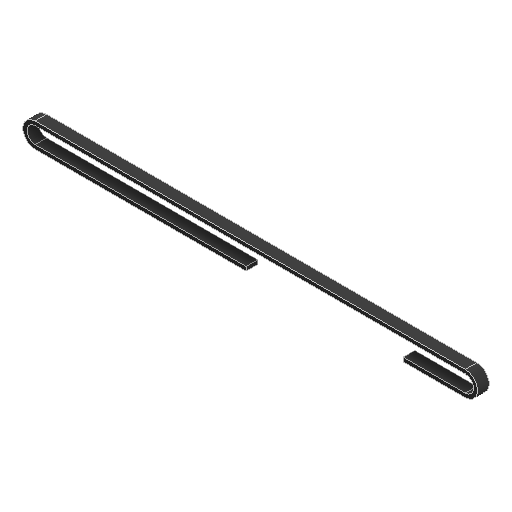
# Autodesk Inventor part: Riemen_T5
Saved by Autodesk Inventor 2022 (Build 260153000, 153)
## iProperties
Created: 2022-10-06
Part Number: Riemen_T5
Material: Gummi
Document SubType Name: Modeling
Designer: alexw
Mass: 23.1241 g
Surface Area: 192.513 cm^2
Volume: 24.8646 cm^3
Density: 0.93 g/cm^3
Appearance: Gummi - Schwarz
Author: alexw
Autodesk Inventor part; units mm, degrees
ref_plane "YZ Plane" through (0, 0, 0) normal (1, 0, 0) x (0, 1, 0)
ref_plane "XZ Plane" through (0, 0, 0) normal (0, 1, 0) x (-1, 0, 0)
ref_plane "XY Plane" through (0, 0, 0) normal (0, 0, 1) x (1, 0, 0)
sketch "Skizze1" plane through (0, 0, 0) normal (0, 0, 1) x (1, 0, 0)
  circle A0 centre (-380.4963, -115.5552) radius 3 construction
  circle A1 centre (-10.4963, -115.5552) radius 3.1 construction
  circle A2 centre (-380.4963, -115.5552) radius 10.57 construction
  circle A3 centre (-10.4963, -115.5552) radius 10.57 construction
  line L0 (-10.4963, -104.9852) -> (-380.4963, -104.9852)
  line L1 (-380.4963, -115.5552) -> (-380.4963, -104.9852) construction
  arc A4 (-380.4963, -104.9852) -> (-380.4963, -126.1252) centre (-380.4963, -115.5552) ccw
  line L2 (-380.4963, -126.1252) -> (-10.4963, -126.1252)
  arc A5 (-10.4963, -126.1252) -> (-10.4963, -104.9852) centre (-10.4963, -115.5552) ccw
  circle A6 centre (-380.4963, -115.5552) radius 7.07 construction
  circle A7 centre (-10.4963, -115.5552) radius 7.07 construction
  line L3 (-10.4963, -122.6252) -> (-380.4963, -122.6252)
  arc A8 (-380.4963, -108.4852) -> (-380.4963, -122.6252) centre (-380.4963, -115.5552) ccw
  line L4 (-380.4963, -108.4852) -> (-10.4963, -108.4852)
  arc A9 (-10.4963, -122.6252) -> (-10.4963, -108.4852) centre (-10.4963, -115.5552) ccw
  line L5 (-198.9963, -126.1252) -> (-198.9963, -122.6252)
  line L6 (-63.9963, -122.6252) -> (-63.9963, -126.1252)
  line L7 (-10.4963, -124.3752) -> (-380.4963, -124.3752) construction
  arc A10 (-380.4963, -106.7352) -> (-380.4963, -124.3752) centre (-380.4963, -115.5552) ccw construction
  line L8 (-380.4963, -106.7352) -> (-10.4963, -106.7352) construction
  arc A11 (-10.4963, -124.3752) -> (-10.4963, -106.7352) centre (-10.4963, -115.5552) ccw construction
  point P0 (0, 0)
  dimension "d0" = 370
  dimension "d1" = 21.14
  dimension "d2" = 21.14
  dimension "d3" = 370
  dimension "d5" = 3.5
  dimension "d8" = 53.5
  dimension "d9" = 181.5
  dimension "d10" = 1.75
  dimension "d11" = 181.5
  dimension "d12" = 370
  dimension "d13" = 53.5
  dimension "d14" = 8.82
  dimension "d15" = 8.82
  dimension "d16" = 14.14
  constraints: 20 point on circle, 18 end point, 10 centre point, 10 tangent, 6 point on line, 4 coincident, 3 perpendicular, 2 concentric, 1 vertical, 3 other
  measures "d0" distance of A1.centre A0.centre
  measures "d1" diameter of A3
  measures "d2" diameter of A2
  measures "d3" distance of A1.centre A0.centre
  measures "d5" radial gap between concentric circles of A3 A7
  measures "d8" distance from line of A1.centre L6
  measures "d9" distance from line of L5 A0.centre
  measures "d10" distance between parallel lines of L2 L7
  measures "d11" distance from line of L7.end L5
  measures "d12" distance of L8.end L8.start
  measures "d13" distance from line of L6 L7.start
  measures "d14" radius of A10
  measures "d15" radius of A11
  measures "d16" diameter of A6
extrude "Extrusion1" add sketch "Skizze1" along normal mid plane 10 contours A5 L2 L6 L3 A9 L4 A8 L5 A4 L0
equation "\"d2\" = d1"
equation "\"d8\" = Riemen_L_UpBottom"
equation "\"d9\" = Riemen_L_BottomUp"
equation "\"d10\" = 0.5 * d4"
equation "\"Bogenlaenge\" = 27.70885"
equation "\"Riemenlaenge\" = d12 + 2 * Bogenlaenge + d13 + d11"
equation "\"Riemen_L_UpBottom\" = 53.5"
equation "\"Riemen_L_BottomUp\" = 181.5"
equation "\"d4\" = 3.5"
